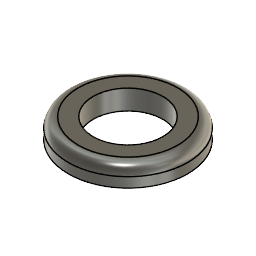
Washer (Autodesk Fusion 360 design; units mm, degrees)
Autodesk Fusion 360 part; units mm, degrees
sketch "Sketch1" plane through (0, 0, 0) normal (0, 0, 1) x (1, 0, 0)
  circle A0 centre (0, 0) radius 9.525
  dimension "d1" = 19.05
  constraint coincident A0.centre origin
  measures "d1" diameter of A0
extrude "Extrude1" add sketch "Sketch1" along normal blind 3.175
fillet "Fillet1" radius 1.5875 1 edges at (-8.8804, -3.4444, 3.175)
sketch "Sketch2" plane through (0, 0, 3.175) normal (0, 0, 1) x (-1, 0, 0)
  circle A0 centre (0, 0) radius 7.9375
  circle A1 centre (0, 0) radius 5.5563
  dimension "d6" = 11.1125
  constraint coincident A0.centre A1.centre
  measures "d6" diameter of A1
extrude "Extrude2" cut sketch "Sketch2" against normal blind 3.175 contours A1
